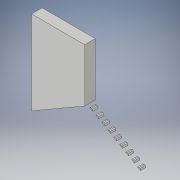
# Autodesk Inventor part: top left door
Saved by Autodesk Inventor 2017 (Build 210142000, 142)
## iProperties
Created: 2018-03-10
Part Number: top left door
Material: Generic
Document SubType Name: Modeling
Designer: Braxton
Density: 1 g/cm^3
Appearance: Default
Author: Braxton
Autodesk Inventor part; units mm, degrees
ref_plane "YZ Plane" through (0, 0, 0) normal (1, 0, 0) x (0, 1, 0)
ref_plane "XZ Plane" through (0, 0, 0) normal (0, 1, 0) x (-1, 0, 0)
ref_plane "XY Plane" through (0, 0, 0) normal (0, 0, 1) x (1, 0, 0)
sketch "Sketch1" plane through (0, 0, 0) normal (0, 0, 1) x (1, 0, 0)
  line L0 (1270, 1270) -> (0, 536.7652)
  line L1 (0, 536.7652) -> (0, 2540)
  line L2 (0, 2540) -> (1270, 2540)
  line L3 (1270, 1270) -> (1270, 2540)
  dimension "d446" = 2003.2348
  constraints: 8 end point, 1 perpendicular
  measures "d446" distance of L0.end L1.end
extrude "door" add sketch "Sketch1" along normal mid plane 254
sketch "Sketch3" plane through (0, 0, 0) normal (0, 0, 1) x (1, 0, 0)
  line L0 (0, 0) -> (0, 536.7652) projected
  line L1 (33.8905, 585.6612) -> (71.1839, 577.8632)
  line L2 (35.592, 557.3142) -> (22.892, 579.3112) construction
  line L3 (11.8934, 572.9612) -> (33.8905, 585.6612)
  line L4 (11.8934, 572.9612) -> (0, 536.7652)
  line L5 (1270, 1270) -> (1270, 0) construction
  line L6 (0, 536.7652) -> (71.1839, 577.8632)
  line L7 (71.1839, 577.8632) -> (108.4774, 570.0652)
  line L8 (108.4774, 570.0652) -> (130.4744, 582.7652)
  line L9 (130.4744, 582.7652) -> (142.3679, 618.9613)
  line L10 (1270, 1270) -> (0, 536.7652) projected
  line L11 (71.1839, 577.8632) -> (142.3679, 618.9613)
  line L12 (106.7759, 598.4123) -> (119.4759, 576.4152) construction
  line L13 (154.2613, 655.1574) -> (142.3679, 618.9613)
  line L14 (154.2613, 655.1574) -> (176.2584, 667.8574)
  line L15 (177.9598, 639.5103) -> (165.2598, 661.5074) construction
  line L16 (176.2584, 667.8574) -> (213.5518, 660.0593)
  line L17 (142.3679, 618.9613) -> (213.5518, 660.0593)
  line L18 (213.5518, 660.0593) -> (250.8452, 652.2613)
  line L19 (250.8452, 652.2613) -> (272.8423, 664.9613)
  line L20 (272.8423, 664.9613) -> (284.7357, 701.1574)
  line L21 (213.5518, 660.0593) -> (284.7357, 701.1574)
  line L22 (249.1438, 680.6084) -> (261.8438, 658.6113) construction
  line L23 (296.6292, 737.3535) -> (284.7357, 701.1574)
  line L24 (296.6292, 737.3535) -> (318.6262, 750.0535)
  line L25 (320.3277, 721.7064) -> (307.6277, 743.7035) construction
  line L26 (318.6262, 750.0535) -> (355.9197, 742.2555)
  line L27 (284.7357, 701.1574) -> (355.9197, 742.2555)
  line L28 (355.9197, 742.2555) -> (393.2131, 734.4575)
  line L29 (393.2131, 734.4575) -> (415.2102, 747.1575)
  line L30 (415.2102, 747.1575) -> (427.1036, 783.3535)
  line L31 (355.9197, 742.2555) -> (427.1036, 783.3535)
  line L32 (391.5116, 762.8045) -> (404.2116, 740.8075) construction
  line L33 (438.997, 819.5496) -> (427.1036, 783.3535)
  line L34 (438.997, 819.5496) -> (460.9941, 832.2496)
  line L35 (462.6956, 803.9026) -> (449.9956, 825.8996) construction
  line L36 (460.9941, 832.2496) -> (498.2875, 824.4516)
  line L37 (427.1036, 783.3535) -> (498.2875, 824.4516)
  line L38 (498.2875, 824.4516) -> (535.581, 816.6536)
  line L39 (535.581, 816.6536) -> (557.578, 829.3536)
  line L40 (557.578, 829.3536) -> (569.4715, 865.5497)
  line L41 (498.2875, 824.4516) -> (569.4715, 865.5497)
  line L42 (533.8795, 845.0006) -> (546.5795, 823.0036) construction
  line L43 (581.3649, 901.7457) -> (569.4715, 865.5497)
  line L44 (581.3649, 901.7457) -> (603.362, 914.4457)
  line L45 (605.0634, 886.0987) -> (592.3634, 908.0957) construction
  line L46 (603.362, 914.4457) -> (640.6554, 906.6477)
  line L47 (569.4715, 865.5497) -> (640.6554, 906.6477)
  line L48 (640.6554, 906.6477) -> (677.9488, 898.8497)
  line L49 (677.9488, 898.8497) -> (699.9459, 911.5497)
  line L50 (699.9459, 911.5497) -> (711.8393, 947.7458)
  line L51 (640.6554, 906.6477) -> (711.8393, 947.7458)
  line L52 (676.2474, 927.1968) -> (688.9474, 905.1997) construction
  line L53 (723.7328, 983.9419) -> (711.8393, 947.7458)
  line L54 (723.7328, 983.9419) -> (745.7298, 996.6419)
  line L55 (747.4313, 968.2948) -> (734.7313, 990.2919) construction
  line L56 (745.7298, 996.6419) -> (783.0233, 988.8439)
  line L57 (711.8393, 947.7458) -> (783.0233, 988.8439)
  line L58 (783.0233, 988.8439) -> (820.3167, 981.0458)
  line L59 (820.3167, 981.0458) -> (842.3138, 993.7458)
  line L60 (842.3138, 993.7458) -> (854.2072, 1029.9419)
  line L61 (783.0233, 988.8439) -> (854.2072, 1029.9419)
  line L62 (818.6152, 1009.3929) -> (831.3152, 987.3958) construction
  line L63 (866.1006, 1066.138) -> (854.2072, 1029.9419)
  line L64 (866.1006, 1066.138) -> (888.0977, 1078.838)
  line L65 (889.7992, 1050.4909) -> (877.0992, 1072.488) construction
  line L66 (888.0977, 1078.838) -> (925.3911, 1071.04)
  line L67 (854.2072, 1029.9419) -> (925.3911, 1071.04)
  line L68 (925.3911, 1071.04) -> (962.6846, 1063.242)
  line L69 (962.6846, 1063.242) -> (984.6816, 1075.942)
  line L70 (984.6816, 1075.942) -> (996.5751, 1112.138)
  line L71 (925.3911, 1071.04) -> (996.5751, 1112.138)
  line L72 (960.9831, 1091.589) -> (973.6831, 1069.592) construction
  line L73 (1008.4685, 1148.3341) -> (996.5751, 1112.138)
  line L74 (1008.4685, 1148.3341) -> (1030.4656, 1161.0341)
  line L75 (1032.167, 1132.6871) -> (1019.467, 1154.6841) construction
  line L76 (1030.4656, 1161.0341) -> (1067.759, 1153.2361)
  line L77 (996.5751, 1112.138) -> (1067.759, 1153.2361)
  line L78 (1067.759, 1153.2361) -> (1105.0525, 1145.4381)
  line L79 (1105.0525, 1145.4381) -> (1127.0495, 1158.1381)
  line L80 (1127.0495, 1158.1381) -> (1138.9429, 1194.3342)
  line L81 (1067.759, 1153.2361) -> (1138.9429, 1194.3342)
  line L82 (1103.351, 1173.7851) -> (1116.051, 1151.7881) construction
  line L83 (1172.8334, 1243.2302) -> (1210.1269, 1235.4322)
  line L84 (1174.5349, 1214.8832) -> (1161.8349, 1236.8802) construction
  line L85 (1150.8364, 1230.5302) -> (1172.8334, 1243.2302)
  line L86 (1150.8364, 1230.5302) -> (1138.9429, 1194.3342)
  line L87 (1138.9429, 1194.3342) -> (1210.1269, 1235.4322)
  line L88 (2528.1066, 572.9612) -> (2506.1095, 585.6612)
  line L89 (2504.408, 557.3142) -> (2517.108, 579.3112) construction
  line L90 (2506.1095, 585.6612) -> (2468.8161, 577.8632)
  line L91 (2540, 536.7652) -> (2468.8161, 577.8632)
  line L92 (2468.8161, 577.8632) -> (2431.5226, 570.0652)
  line L93 (2431.5226, 570.0652) -> (2409.5256, 582.7652)
  line L94 (2409.5256, 582.7652) -> (2397.6321, 618.9613)
  line L95 (2540, 536.7652) -> (1270, 1270)
  line L96 (2468.8161, 577.8632) -> (2397.6321, 618.9613)
  line L97 (2433.2241, 598.4123) -> (2420.5241, 576.4152) construction
  line L98 (2267.1577, 664.9613) -> (2255.2643, 701.1574)
  line L99 (2289.1548, 652.2613) -> (2267.1577, 664.9613)
  line L100 (2290.8562, 680.6084) -> (2278.1562, 658.6113) construction
  line L101 (2326.4482, 660.0593) -> (2255.2643, 701.1574)
  line L102 (2326.4482, 660.0593) -> (2289.1548, 652.2613)
  line L103 (2363.7416, 667.8574) -> (2326.4482, 660.0593)
  line L104 (2362.0402, 639.5103) -> (2374.7402, 661.5074) construction
  line L105 (2385.7387, 655.1574) -> (2363.7416, 667.8574)
  line L106 (2385.7387, 655.1574) -> (2397.6321, 618.9613)
  line L107 (2397.6321, 618.9613) -> (2326.4482, 660.0593)
  line L108 (2124.7898, 747.1575) -> (2112.8964, 783.3535)
  line L109 (2146.7869, 734.4575) -> (2124.7898, 747.1575)
  line L110 (2148.4884, 762.8045) -> (2135.7884, 740.8075) construction
  line L111 (2184.0803, 742.2555) -> (2112.8964, 783.3535)
  line L112 (2184.0803, 742.2555) -> (2146.7869, 734.4575)
  line L113 (2221.3738, 750.0535) -> (2184.0803, 742.2555)
  line L114 (2219.6723, 721.7064) -> (2232.3723, 743.7035) construction
  line L115 (2243.3708, 737.3535) -> (2221.3738, 750.0535)
  line L116 (2243.3708, 737.3535) -> (2255.2643, 701.1574)
  line L117 (2255.2643, 701.1574) -> (2184.0803, 742.2555)
  line L118 (1982.422, 829.3536) -> (1970.5285, 865.5497)
  line L119 (2004.419, 816.6536) -> (1982.422, 829.3536)
  line L120 (2006.1205, 845.0006) -> (1993.4205, 823.0036) construction
  line L121 (2041.7125, 824.4516) -> (1970.5285, 865.5497)
  line L122 (2041.7125, 824.4516) -> (2004.419, 816.6536)
  line L123 (2079.0059, 832.2496) -> (2041.7125, 824.4516)
  line L124 (2077.3044, 803.9026) -> (2090.0044, 825.8996) construction
  line L125 (2101.003, 819.5496) -> (2079.0059, 832.2496)
  line L126 (2101.003, 819.5496) -> (2112.8964, 783.3535)
  line L127 (2112.8964, 783.3535) -> (2041.7125, 824.4516)
  line L128 (1840.0541, 911.5497) -> (1828.1607, 947.7458)
  line L129 (1862.0512, 898.8497) -> (1840.0541, 911.5497)
  line L130 (1863.7526, 927.1968) -> (1851.0526, 905.1997) construction
  line L131 (1899.3446, 906.6477) -> (1828.1607, 947.7458)
  line L132 (1899.3446, 906.6477) -> (1862.0512, 898.8497)
  line L133 (1936.638, 914.4457) -> (1899.3446, 906.6477)
  line L134 (1934.9366, 886.0987) -> (1947.6366, 908.0957) construction
  line L135 (1958.6351, 901.7457) -> (1936.638, 914.4457)
  line L136 (1958.6351, 901.7457) -> (1970.5285, 865.5497)
  line L137 (1970.5285, 865.5497) -> (1899.3446, 906.6477)
  line L138 (1697.6862, 993.7458) -> (1685.7928, 1029.9419)
  line L139 (1719.6833, 981.0458) -> (1697.6862, 993.7458)
  line L140 (1721.3848, 1009.3929) -> (1708.6848, 987.3958) construction
  line L141 (1756.9767, 988.8439) -> (1685.7928, 1029.9419)
  line L142 (1756.9767, 988.8439) -> (1719.6833, 981.0458)
  line L143 (1794.2702, 996.6419) -> (1756.9767, 988.8439)
  line L144 (1792.5687, 968.2948) -> (1805.2687, 990.2919) construction
  line L145 (1816.2672, 983.9419) -> (1794.2702, 996.6419)
  line L146 (1816.2672, 983.9419) -> (1828.1607, 947.7458)
  line L147 (1828.1607, 947.7458) -> (1756.9767, 988.8439)
  line L148 (1555.3184, 1075.942) -> (1543.4249, 1112.138)
  line L149 (1577.3154, 1063.242) -> (1555.3184, 1075.942)
  line L150 (1579.0169, 1091.589) -> (1566.3169, 1069.592) construction
  line L151 (1614.6089, 1071.04) -> (1543.4249, 1112.138)
  line L152 (1614.6089, 1071.04) -> (1577.3154, 1063.242)
  line L153 (1651.9023, 1078.838) -> (1614.6089, 1071.04)
  line L154 (1650.2008, 1050.4909) -> (1662.9008, 1072.488) construction
  line L155 (1673.8994, 1066.138) -> (1651.9023, 1078.838)
  line L156 (1673.8994, 1066.138) -> (1685.7928, 1029.9419)
  line L157 (1685.7928, 1029.9419) -> (1614.6089, 1071.04)
  line L158 (1412.9505, 1158.1381) -> (1401.0571, 1194.3342)
  line L159 (1434.9475, 1145.4381) -> (1412.9505, 1158.1381)
  line L160 (1436.649, 1173.7851) -> (1423.949, 1151.7881) construction
  line L161 (1472.241, 1153.2361) -> (1401.0571, 1194.3342)
  line L162 (1472.241, 1153.2361) -> (1434.9475, 1145.4381)
  line L163 (1509.5344, 1161.0341) -> (1472.241, 1153.2361)
  line L164 (1507.833, 1132.6871) -> (1520.533, 1154.6841) construction
  line L165 (1531.5315, 1148.3341) -> (1509.5344, 1161.0341)
  line L166 (1531.5315, 1148.3341) -> (1543.4249, 1112.138)
  line L167 (1543.4249, 1112.138) -> (1472.241, 1153.2361)
  line L168 (1389.1636, 1230.5302) -> (1401.0571, 1194.3342)
  line L169 (1365.4651, 1214.8832) -> (1378.1651, 1236.8802) construction
  line L170 (1389.1636, 1230.5302) -> (1367.1666, 1243.2302)
  line L171 (1401.0571, 1194.3342) -> (1329.8731, 1235.4322)
  line L172 (1367.1666, 1243.2302) -> (1329.8731, 1235.4322)
  line L173 (2540, 0) -> (2540, 536.7652) projected
  line L174 (2528.1066, 572.9612) -> (2540, 536.7652)
  dimension "d282" = 25.4
  dimension "d283" = 25.4
  dimension "d284" = 38.1
  dimension "d285" = 38.1
  dimension "d350" = 38.1
  dimension "d351" = 25.4
  dimension "d352" = 38.1
  dimension "d353" = 138.19
  dimension "d356" = 138.19
  dimension "d358" = 25.4
  dimension "d359" = 25.4
  dimension "d360" = 25.4
  dimension "d361" = 38.1
  dimension "d362" = 38.1
  dimension "d363" = 38.1
  dimension "d364" = 25.4
  dimension "d365" = 38.1
  dimension "d366" = 138.19
  dimension "d367" = 138.19
  dimension "d368" = 25.4
  dimension "d369" = 25.4
  dimension "d370" = 25.4
  dimension "d371" = 38.1
  dimension "d372" = 38.1
  dimension "d373" = 38.1
  dimension "d374" = 25.4
  dimension "d375" = 38.1
  dimension "d376" = 138.19
  dimension "d377" = 138.19
  dimension "d378" = 25.4
  dimension "d379" = 25.4
  dimension "d380" = 25.4
  dimension "d381" = 38.1
  dimension "d382" = 38.1
  dimension "d383" = 38.1
  dimension "d384" = 25.4
  dimension "d385" = 38.1
  dimension "d386" = 138.19
  dimension "d387" = 138.19
  dimension "d388" = 25.4
  dimension "d389" = 25.4
  dimension "d390" = 25.4
  dimension "d391" = 38.1
  dimension "d392" = 38.1
  dimension "d393" = 38.1
  dimension "d394" = 25.4
  dimension "d395" = 38.1
  dimension "d396" = 138.19
  dimension "d397" = 138.19
  dimension "d398" = 25.4
  dimension "d399" = 25.4
  dimension "d400" = 25.4
  dimension "d401" = 38.1
  dimension "d402" = 38.1
  dimension "d403" = 38.1
  dimension "d404" = 25.4
  dimension "d405" = 38.1
  dimension "d406" = 138.19
  dimension "d407" = 138.19
  dimension "d408" = 25.4
  dimension "d409" = 25.4
  dimension "d410" = 25.4
  dimension "d411" = 38.1
  dimension "d412" = 38.1
  constraints: 344 end point, 86 symmetric about line, 25 midpoint, 18 perpendicular, 13 collinear, 1 vertical
  measures "d282" distance of L2.start L2.end
  measures "d283" distance of L4.start L3.end
  measures "d284" distance of L0.end L4.start
  measures "d285" distance of L3.end L1.end
  measures "d350" distance of L1.end L7.end
  measures "d351" distance of L7.end L8.end
  measures "d352" distance of L9.end L8.end
  measures "d353" angle of L3 L4
  measures "d356" angle of L8 L7
  measures "d358" distance of L12.start L12.end
  measures "d359" distance of L15.start L15.end
  measures "d360" distance of L14.start L16.start
  measures "d361" distance of L9.end L14.start
  measures "d362" distance of L16.start L21.start
  measures "d363" distance of L21.start L19.start
  measures "d364" distance of L19.start L20.start
  measures "d365" distance of L20.end L20.start
  measures "d366" angle of L14 L13
  measures "d367" angle of L19 L18
  measures "d368" distance of L22.start L22.end
  measures "d369" distance of L25.start L25.end
  measures "d370" distance of L24.start L26.start
  measures "d371" distance of L20.end L24.start
  measures "d372" distance of L26.start L31.start
  measures "d373" distance of L31.start L29.start
  measures "d374" distance of L29.start L30.start
  measures "d375" distance of L30.end L30.start
  measures "d376" angle of L24 L23
  measures "d377" angle of L29 L28
  measures "d378" distance of L32.start L32.end
  measures "d379" distance of L35.start L35.end
  measures "d380" distance of L34.start L36.start
  measures "d381" distance of L30.end L34.start
  measures "d382" distance of L36.start L41.start
  measures "d383" distance of L41.start L39.start
  measures "d384" distance of L39.start L40.start
  measures "d385" distance of L40.end L40.start
  measures "d386" angle of L34 L33
  measures "d387" angle of L39 L38
  measures "d388" distance of L42.start L42.end
  measures "d389" distance of L45.start L45.end
  measures "d390" distance of L44.start L46.start
  measures "d391" distance of L40.end L44.start
  measures "d392" distance of L46.start L51.start
  measures "d393" distance of L51.start L49.start
  measures "d394" distance of L49.start L50.start
  measures "d395" distance of L50.end L50.start
  measures "d396" angle of L44 L43
  measures "d397" angle of L49 L48
  measures "d398" distance of L52.start L52.end
  measures "d399" distance of L55.start L55.end
  measures "d400" distance of L54.start L56.start
  measures "d401" distance of L50.end L54.start
  measures "d402" distance of L56.start L61.start
  measures "d403" distance of L61.start L59.start
  measures "d404" distance of L59.start L60.start
  measures "d405" distance of L60.end L60.start
  measures "d406" angle of L54 L53
  measures "d407" angle of L59 L58
  measures "d408" distance of L62.start L62.end
  measures "d409" distance of L65.start L65.end
  measures "d410" distance of L64.start L66.start
  measures "d411" distance of L60.end L64.start
  measures "d412" distance of L66.start L71.start
extrude "connection give" add sketch "Sketch3" along normal mid plane 127 contours L86 L85 L83 L10 | L73 L74 L76 L10 | L63 L64 L66 L10 | L53 L54 L56 L10 | L43 L44 L46 L10 | L33 L34 L36 L10 | L23 L24 L26 L10 | L13 L14 L16 L10 | L1 L6 L4 L3 | L174 L91 L90 L88 | L95 L172 L170 L168 | L95 L163 L165 L166 | L95 L153 L155 L156 | L95 L143 L145 L146 | L95 L133 L135 L136 | L95 L123 L125 L126 | L95 L113 L115 L116 | L95 L103 L105 L106
extrude "connection receive" cut sketch "Sketch3" along normal mid plane 127 contours L10 L80 L79 L78 | L10 L70 L69 L68 | L10 L60 L59 L58 | L10 L50 L49 L48 | L10 L40 L39 L38 | L10 L30 L29 L28 | L10 L20 L19 L18 | L10 L9 L8 L7 | L162 L159 L158 L95 | L152 L149 L148 L95 | L142 L139 L138 L95 | L132 L129 L128 L95 | L122 L119 L118 L95 | L112 L109 L108 L95 | L102 L99 L98 L95 | L92 L93 L94 L95
body "Solid1"
